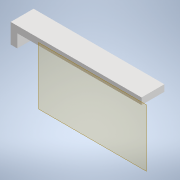
# Autodesk Inventor part: fence
Saved by Autodesk Inventor 2020 (Build 240168000, 168)
## iProperties
Created: 2019-05-07
Part Number: fence
Material: Generic
Document SubType Name: Modeling
Designer: erwin
Density: 1 g/cm^3
Appearance: Default
Author: erwin
Autodesk Inventor part; units mm, degrees
ref_plane "YZ Plane" through (0, 0, 0) normal (1, 0, 0) x (0, 1, 0)
ref_plane "XZ Plane" through (0, 0, 0) normal (0, 1, 0) x (-1, 0, 0)
ref_plane "Work Plane1" through (0, 0, 0) normal (0, 0, 1) x (1, 0, 0)
sketch "Sketch1" plane through (0, 0, 0) normal (0, 0, 1) x (1, 0, 0)
  line L0 (0, 0) -> (0, -15.5) projected
  line L1 (0, -15.5) -> (30, -15.5) projected
  line L2 (30, -0.5) -> (30, -15.5) projected
  line L3 (0, -0.5) -> (30, -0.5) projected
  line L4 (30, -0.5) -> (-10, -0.5)
  line L5 (-10, -0.5) -> (-10, 1.5)
  line L6 (-10, 1.5) -> (30, 1.5)
  line L7 (30, 1.5) -> (30, -0.5)
  point P0 (0, -0.5)
  dimension "d0" = 40
  dimension "d1" = 2
  constraints: 8 end point, 2 parallel, 1 horizontal, 1 perpendicular, 1 other
  measures "d0" distance of L5.end L6.end
  measures "d1" distance of L4.end L5.end
extrude "Extrusion1" add sketch "Sketch1" against normal up to surface (7 mm away) contours L4 L5 L6 L7 L3
ref_plane "Work Plane2" through (0, -16, -7) normal (0, -1, 0) x (1, 0, 0)
move faces "Move1" translate (0, -0.5, 0) faces at (16.6667, 1.5, -2.3333)
sketch "Sketch3" plane through (-10, -0.5, 0) normal (0, -1, 0) x (1, 0, 0)
  line L0 (40, 0) -> (0, 0) projected
  line L1 (0, 0) -> (-2, 0)
  line L2 (-2, 0) -> (-2, -7)
  line L3 (-2, -7) -> (0, -7)
  line L4 (0, -7) -> (0, 0)
  point P0 (10, 0)
  dimension "d19" = 2
  constraints: 8 end point, 2 parallel, 1 horizontal, 1 perpendicular
  measures "d19" distance of L3.end L2.end
extrude "Extrusion3" add sketch "Sketch3" along normal blind 7 and the other way blind 7
body "Solid1"
